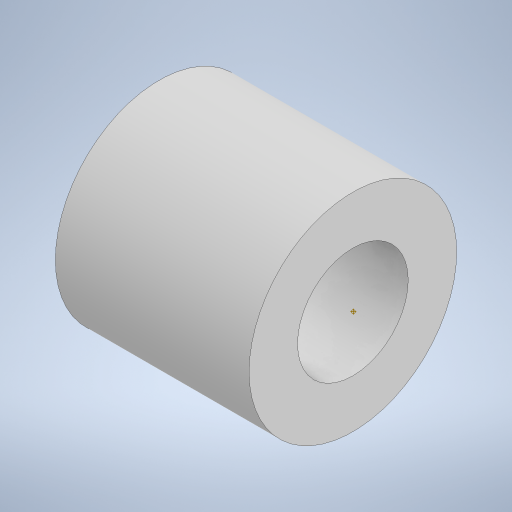
# Autodesk Inventor part: Embouts
Saved by Autodesk Inventor 2023.2 (Build 272271030, 271C)
## iProperties
Created: 2023-03-02
Part Number: Embouts
Material: Generic
Document SubType Name: Modeling
Designer: Luis Valente
Density: 1 g/cm^3
Appearance: Default
Author: Luis Valente
Autodesk Inventor part; units mm, degrees
ref_plane "Work Plane9" through (86, 0, 0) normal (-1, 0, 0) x (0, 0, 1)
ref_plane "Work Plane3" through (-100, 0, 0) normal (-1, 0, 0) x (0, 0, 1)
sketch "Sketch8" plane through (-100, 0, 0) normal (-1, 0, 0) x (0, 0, 1)
  circle A0 centre (0, 0) radius 7.5
  dimension "d21" = 15
  constraints: 1 centre point, 1 coincident
  measures "d21" diameter of A0
extrude "Extrusion4" add sketch "Sketch8" against normal blind 14
ref_plane "Work Plane4" through (86, 0, 0) normal (-1, 0, 0) x (0, 0, 1)
hole "Hole2" at (-86, 0, 0) direction (-1, 0, 0) diameter 8 depth 10 tip angle 120
body "Solid2"
